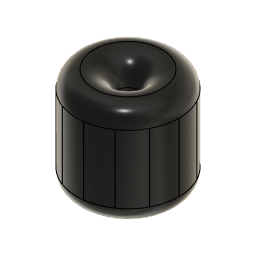
bodyyyy_v3 (Autodesk Fusion 360 archive; units mm, degrees)
design "parachute"
Autodesk Fusion 360 part; units mm, degrees
cylinder "CylinderPrimitive1" add diameter 30 height 30 placed x (1, 0, 0) y (0, 1, 0) z (0, 0, 1) at (0, 0, 0)
sketch "Sketch2" plane through (0, 0, 30) normal (0, 0, 1) x (-1, 0, 0)
  circle A0 centre (0, 0) radius 15
  circle A1 centre (0, 0) radius 3.25
  dimension "d3" = 6.5
  constraint concentric A0 A1
  measures "d3" diameter of A1
extrude "Extrude1" cut sketch "Sketch2" against normal blind 90 contours A1
fillet "Fillet1" radius 5 2 edges at (-13.9849, -5.4242, 30) (-13.9849, 5.4242, 0)
fillet "Fillet2" radius 7 2 edges at (3.0301, -1.1753, 30) (3.0301, 1.1753, 0)
ref_plane "WorkPlane1" through (15, 0, 15.9859) normal (1, 0, 0) x (0, -1, 0)
sketch "Sketch3" plane through (15, 0, 15.9859) normal (1, 0, 0) x (0, 1, 0)
  line L0 (0, 9) -> (0, -11)
  constraint vertical L0
extrude "Extrude2" cut sketch "Sketch3" against normal blind 0.0001 thin wall 1 on the right open curves L0
pattern_circular "C-Pattern1" count 13 over 360 about axis through (0, 0, 1.75) along (0, 0, 1) of "Extrude2"
